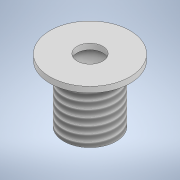
# Autodesk Inventor part: Tapa
Saved by Autodesk Inventor 2022.2 (Build 262287000, 287)
## iProperties
Created: 2022-06-18
Part Number: Tapa
Material: Generic
Document SubType Name: Modeling
Designer: Usuario
Density: 1 g/cm^3
Appearance: Default
Author: Usuario
Autodesk Inventor part; units mm, degrees
ref_plane "YZ Plane" through (0, 0, 0) normal (1, 0, 0) x (0, 1, 0)
ref_plane "XZ Plane" through (0, 0, 0) normal (0, 1, 0) x (-1, 0, 0)
ref_plane "XY Plane" through (0, 0, 0) normal (0, 0, 1) x (1, 0, 0)
sketch "Sketch1" plane through (0, 0, 0) normal (0, 1, 0) x (-1, 0, 0)
  circle A0 centre (0, 0) radius 9.15
  circle A1 centre (0, 0) radius 7.45
  dimension "d0" = 18.3
  dimension "d4" = 1.7
  constraints: 2 centre point, 1 coincident
  measures "d0" diameter of A0
  measures "d4" radial gap between concentric circles of A0 A1
extrude "Extrusion2" add sketch "Sketch1" along normal blind 20
sketch "Sketch2" plane through (0, 20, 0) normal (0, 1, 0) x (1, 0, 0)
  circle A0 centre (0, 0) radius 14
  circle A1 centre (0, 0) radius 4.5
  dimension "d7" = 28
  dimension "d12" = 9
  constraints: 2 centre point, 2 coincident
  measures "d7" diameter of A0
  measures "d12" diameter of A1
extrude "Extrusion3" add sketch "Sketch2" along normal blind 2 contours A0 | A1
thread "Thread1" size "M20x2.5" class "6g" standard "ANSI Metric M Profile" full length
sketch "Sketch3" plane through (0, 22, 0) normal (0, 1, 0) x (1, 0, 0)
  circle A0 centre (0, 0) radius 4.5
  dimension "d13" = 9
  constraints: 1 centre point, 1 coincident
  measures "d13" diameter of A0
extrude "Extrusion4" cut sketch "Sketch3" against normal through all
body "Solid2"
